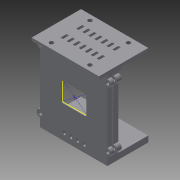
# Autodesk Inventor part: Nikon Base 02
Saved by Autodesk Inventor 2013 (Build 170138000, 138)
## iProperties
Created: 2014-04-13
Part Number: Nikon Base 02
Material: Generic
Document SubType Name: Modeling
Designer: spichelh
Density: 1 g/cm^3
Author: spichelh
Autodesk Inventor part; units mm, degrees
ref_plane "YZ Plane" through (0, 0, 0) normal (1, 0, 0) x (0, 1, 0)
ref_plane "XZ Plane" through (0, 0, 0) normal (0, 1, 0) x (-1, 0, 0)
ref_plane "XY Plane" through (0, 0, 0) normal (0, 0, 1) x (1, 0, 0)
sketch "Sketch1" plane through (0, 0, 0) normal (0, 0, 1) x (1, 0, 0)
  line L0 (55.88, 58.53) -> (0, 58.53)
  circle A0 centre (0, 3) radius 1.5
  arc A1 (0, 6) -> (0, 0) centre (0, 3) ccw
  circle A2 centre (0, 52.53) radius 1.5
  arc A3 (0, 55.53) -> (0, 49.53) centre (0, 52.53) ccw
  line L1 (27.94, 5) -> (27.94, 58.53) construction
  circle A4 centre (55.88, 3) radius 1.5
  arc A5 (55.88, 0) -> (55.88, 6) centre (55.88, 3) ccw
  circle A6 centre (55.88, 52.53) radius 1.5
  arc A7 (55.88, 49.53) -> (55.88, 55.53) centre (55.88, 52.53) ccw
  line L2 (55.88, 6) -> (55.88, 49.53)
  line L3 (55.88, 55.53) -> (55.88, 58.53)
  line L4 (0, 58.53) -> (0, 55.53)
  line L5 (0, 49.53) -> (0, 6)
  line L6 (52.88, 56.53) -> (3, 56.53)
  line L7 (0, 0) -> (0, 6) construction
  line L8 (55.88, 0) -> (55.88, 6) construction
  line L9 (0, 0) -> (0, -7)
  line L10 (0, -7) -> (55.88, -7)
  line L11 (55.88, -7) -> (55.88, 0)
  line L12 (50.88, 56.34) -> (5, 56.34) construction
  line L13 (3, -2.5) -> (52.88, -2.5)
  line L14 (3, 56.53) -> (3, -2.5)
  line L15 (52.88, -2.5) -> (52.88, 56.53)
  dimension "d0" = 55.88
  dimension "d2" = 3
  dimension "d3" = 6
  dimension "d4" = 3
  dimension "d5" = 6
  dimension "d6" = 49.53
  dimension "d8" = 3
  dimension "d14" = 2
  dimension "d16" = 7
  dimension "d17" = 7
  dimension "d78" = 3
  dimension "d79" = 3
  dimension "d214" = 4.5
  dimension "d215" = 3
  constraints: 30 end point, 9 parallel, 8 centre point, 8 point on circle, 5 coincident, 4 symmetric about line, 3 midpoint, 3 perpendicular, 1 collinear, 1 point on line, 4 other
  measures "d0" distance of L7.start L8.start
  measures "d2" diameter of A0
  measures "d3" diameter of A1
  measures "d4" diameter of A2
  measures "d5" diameter of A3
  measures "d6" distance of A0.centre A2.centre
  measures "d8" distance of A0.centre L7.start
  measures "d14" distance between parallel lines of L0 L6
  measures "d16" distance of L7.start L9.end
  measures "d17" distance of L10.end L8.start
  measures "d78" distance between parallel lines of L15 L2
  measures "d79" distance between parallel lines of L5 L14
  measures "d214" distance between parallel lines of L10 L13
  measures "d215" distance of L0.end L4.end
extrude "Extrusion1" add sketch "Sketch1" along normal blind 9
sketch "Sketch14" plane through (0, 0, 9) normal (0, 0, 1) x (1, 0, 0)
  line L0 (3, 56.53) -> (52.88, 56.53)
  line L1 (52.88, 56.53) -> (52.88, -2.5)
  line L2 (52.88, -2.5) -> (3, -2.5)
  line L3 (3, -2.5) -> (3, 56.53)
  circle A0 centre (27.94, 27.765) radius 23
  line L4 (27.94, 56.53) -> (27.94, -2.5) construction
  line L5 (50.88, 56.34) -> (5, 56.34) construction
  line L6 (-22.86, -0.81) -> (78.74, -0.81) construction
  line L7 (-22.86, 56.34) -> (-22.86, -0.81) construction
  line L8 (78.74, -0.81) -> (78.74, 56.34) construction
  line L9 (78.74, 27.765) -> (-22.86, 27.765) construction
  dimension "d96" = 46
  constraints: 12 end point, 5 midpoint, 2 parallel, 1 centre point, 1 horizontal, 1 perpendicular, 1 point on line
  measures "d96" diameter of A0
extrude "Extrusion14" add sketch "Sketch14" against normal blind 2
sketch "Sketch17" plane through (0, 0, 7) normal (0, 0, -1) x (-1, 0, 0)
  circle A0 centre (-27.94, 27.765) radius 23 construction
  line L0 (-37.34, 35.815) -> (-18.54, 35.815)
  line L1 (-17.54, 34.815) -> (-17.54, 20.715)
  line L2 (-18.54, 19.715) -> (-37.34, 19.715)
  line L3 (-38.34, 20.715) -> (-38.34, 34.815)
  line L4 (-17.54, 35.815) -> (-38.34, 19.715) construction
  line L5 (-17.54, 19.715) -> (-38.34, 35.815) construction
  circle A1 centre (-27.94, 27.765) radius 23
  arc A2 (-37.34, 35.815) -> (-38.34, 34.815) centre (-37.34, 34.815) ccw
  arc A3 (-38.34, 20.715) -> (-37.34, 19.715) centre (-37.34, 20.715) ccw
  arc A4 (-18.54, 19.715) -> (-17.54, 20.715) centre (-18.54, 20.715) ccw
  arc A5 (-17.54, 34.815) -> (-18.54, 35.815) centre (-18.54, 34.815) ccw
  point P0 (0, 0)
  dimension "d111" = 20.8
  dimension "d112" = 16.1
  dimension "d115" = 1
  constraints: 12 end point, 8 point on circle, 8 point on line, 8 tangent, 5 centre point, 4 equal radius, 2 midpoint, 2 parallel, 1 coincident, 1 horizontal, 1 perpendicular
  measures "d111" distance of L5.start L4.end
  measures "d112" distance of L4.start L5.start
  measures "d115" radius of A2
extrude "Extrusion17" add sketch "Sketch17" against normal blind 2
sketch "Sketch26" plane through (0, 6, 0) normal (-1, 0, 0) x (0, 0, 1)
  line L0 (0, 0) -> (0, 43.53) projected
  line L1 (-1, 50.34) -> (0, 50.34) construction
  line L2 (-1, -6.81) -> (0, -6.81) construction
  line L3 (4, -6.81) -> (6, -6.81)
  line L4 (6, -6.81) -> (6, 50.34)
  line L5 (6, 50.34) -> (4, 50.34)
  line L6 (4, 50.34) -> (4, -6.81)
  point P0 (0, -6)
  dimension "d140" = 2
  dimension "d141" = 4
  constraints: 8 end point, 2 collinear, 2 parallel, 1 horizontal, 1 perpendicular
  measures "d140" distance of L5.end L4.end
  measures "d141" distance between parallel lines of L0 L6
extrude "Extrusion26" cut sketch "Sketch26" along normal blind 3 and the other way blind 2
sketch "Sketch27" plane through (55.88, 6, 0) normal (1, 0, 0) x (0, 0, -1)
  line L0 (1, -6.81) -> (0, -6.81) construction
  line L1 (1, 50.34) -> (0, 50.34) construction
  line L2 (-4, 50.34) -> (-6, 50.34)
  line L3 (-6, 50.34) -> (-6, -6.81)
  line L4 (-6, -6.81) -> (-4, -6.81)
  line L5 (-4, -6.81) -> (-4, 50.34)
  line L6 (0, -6) -> (0, -13) construction
  dimension "d146" = 2
  dimension "d147" = 4
  constraints: 8 end point, 2 collinear, 2 parallel, 1 horizontal, 1 perpendicular
  measures "d146" distance of L4.end L3.end
  measures "d147" distance between parallel lines of L6 L5
extrude "Extrusion27" cut sketch "Sketch27" against normal blind 1.5 and the other way blind 3
sketch "Sketch32" plane through (0, 0, 0) normal (0, 0, -1) x (-1, 0, 0)
  line L0 (-55.88, -7) -> (0, -7)
  line L1 (0, -7) -> (0, -2)
  line L2 (0, -2) -> (-55.88, -2)
  line L3 (-55.88, -2) -> (-55.88, -7)
  dimension "d180" = 5
  dimension "d206" = 55.88
  constraints: 8 end point, 2 parallel, 1 horizontal, 1 perpendicular
  measures "d180" distance between parallel lines of L0 L2
  measures "d206" distance of L0.start L0.end
extrude "Extrusion32" add sketch "Sketch32" along normal blind 25 and the other way blind 1.5
sketch "Sketch35" plane through (0, -7, 9) normal (0, -1, 0) x (1, 0, 0)
  line L0 (55.88, -34) -> (0, -34) projected
  line L1 (0, -34) -> (55.88, 0) construction
  line L2 (55.88, -34) -> (0, 0) construction
  line L3 (27.94, -17) -> (27.94, -24.0701) construction
  circle A0 centre (27.94, -27) radius 3.175
  circle A1 centre (27.94, -15) radius 3.175
  point P0 (0, -9)
  dimension "d194" = 6.35
  dimension "d195" = 10
  dimension "d196" = 6.35
  dimension "d197" = 2
  constraints: 6 end point, 2 centre point, 2 point on line, 1 midpoint, 1 perpendicular
  measures "d194" diameter of A0
  measures "d195" distance of L3.start A0.centre
  measures "d196" diameter of A1
  measures "d197" distance of L3.start A1.centre
extrude "Extrusion34" cut sketch "Sketch35" against normal blind 10
sketch "Sketch37" plane through (52.88, -2, 0) normal (0, 1, 0) x (1, 0, 0)
  line L0 (-49.88, -1.5) -> (-49.88, 0) projected
  line L1 (0, -1.5) -> (-49.88, -1.5) projected
  line L2 (0, -1.5) -> (-49.88, -1.5)
  line L3 (-49.88, -1.5) -> (-49.88, 0)
  line L4 (-49.88, 0) -> (0, 0)
  line L5 (0, 0) -> (0, -1.5)
  constraints: 8 end point, 2 parallel, 1 horizontal, 1 perpendicular
extrude "Extrusion36" add sketch "Sketch37" along normal blind 3
sketch "Sketch38" plane through (0, 0, 7) normal (0, 0, -1) x (-1, 0, 0)
  arc A0 (-38.34, 20.715) -> (-37.34, 19.715) centre (-37.34, 20.715) ccw projected
  line L0 (-38.34, 20.715) -> (-38.34, 34.815) projected
  arc A1 (-37.34, 35.815) -> (-38.34, 34.815) centre (-37.34, 34.815) ccw projected
  line L1 (-37.34, 35.815) -> (-18.54, 35.815) projected
  arc A2 (-17.54, 34.815) -> (-18.54, 35.815) centre (-18.54, 34.815) ccw projected
  line L2 (-17.54, 34.815) -> (-17.54, 20.715) projected
  arc A3 (-18.54, 19.715) -> (-17.54, 20.715) centre (-18.54, 20.715) ccw projected
  line L3 (-18.54, 19.715) -> (-37.34, 19.715) projected
  line L4 (-18.54, 34.815) -> (-37.34, 20.715) construction
  line L5 (-18.54, 20.715) -> (-37.34, 34.815) construction
  line L6 (-45.055, 44.88) -> (-10.825, 44.88)
  line L7 (-10.825, 44.88) -> (-10.825, 10.65)
  line L8 (-10.825, 10.65) -> (-45.055, 10.65)
  line L9 (-45.055, 10.65) -> (-45.055, 44.88)
  line L10 (-10.825, 10.65) -> (-45.055, 44.88) construction
  line L11 (-45.055, 10.65) -> (-10.825, 44.88) construction
  point P0 (0, 0)
  point P1 (-27.94, 27.765)
  dimension "d209" = 34.23
  dimension "d211" = 34.23
  constraints: 16 end point, 3 midpoint, 2 parallel, 1 horizontal, 1 perpendicular
  measures "d209" distance of L8.end L6.start
  measures "d211" distance of L6.start L6.end
extrude "Extrusion37" cut sketch "Sketch38" against normal blind 1
sketch "Sketch39" plane through (0, 0, 8) normal (0, 0, -1) x (-1, 0, 0)
  line L0 (-37.34, 19.715) -> (-18.54, 19.715) projected
  arc A0 (-38.34, 20.715) -> (-37.34, 19.715) centre (-37.34, 20.715) ccw projected
  line L1 (-38.34, 34.815) -> (-38.34, 20.715) projected
  arc A1 (-37.34, 35.815) -> (-38.34, 34.815) centre (-37.34, 34.815) ccw projected
  line L2 (-18.54, 35.815) -> (-37.34, 35.815) projected
  arc A2 (-17.54, 34.815) -> (-18.54, 35.815) centre (-18.54, 34.815) ccw projected
  line L3 (-17.54, 20.715) -> (-17.54, 34.815) projected
  arc A3 (-18.54, 19.715) -> (-17.54, 20.715) centre (-18.54, 20.715) ccw projected
  line L4 (-45.055, 44.88) -> (-10.825, 44.88) projected
  line L5 (-45.055, 10.65) -> (-45.055, 44.88) projected
  line L6 (-10.825, 10.65) -> (-45.055, 10.65) projected
  line L7 (-10.825, 44.88) -> (-10.825, 10.65) projected
  line L8 (-18.54, 34.815) -> (-37.34, 20.715) construction
  line L9 (-37.34, 34.815) -> (-18.54, 20.715) construction
  point P0 (0, 0)
  point P1 (-27.94, 27.765)
  constraints: 4 end point, 1 midpoint
sketch "Sketch40" plane through (0, 0, 9) normal (0, 0, 1) x (1, 0, 0)
  line L0 (0, 58.53) -> (55.88, 58.53)
  line L1 (55.88, 58.53) -> (55.88, 61.03)
  line L2 (55.88, 61.03) -> (0, 61.03)
  line L3 (0, 61.03) -> (0, 58.53)
  dimension "d216" = 2.5
  dimension "d217" = 55.88
  constraints: 8 end point, 2 parallel, 1 horizontal, 1 perpendicular
  measures "d216" distance of L2.end L0.start
  measures "d217" distance between parallel lines of L3 L1
extrude "Extrusion38" add sketch "Sketch40" along normal blind 7 and the other way blind 34
sketch "Sketch43" plane through (0, 61.03, 16) normal (0, 1, 0) x (1, 0, 0)
  line L0 (52.88, 24) -> (3, 24)
  line L1 (3, 29) -> (3, 24)
  line L2 (52.88, 29) -> (3, 29)
  line L3 (52.88, 29) -> (52.88, 24)
  line L4 (12, 30) -> (14, 30)
  line L5 (14, 30) -> (14, 25)
  line L6 (14, 25) -> (12, 25)
  line L7 (12, 25) -> (12, 30)
  line L8 (17, 30) -> (19, 30)
  line L9 (19, 30) -> (19, 25)
  line L10 (19, 25) -> (17, 25)
  line L11 (17, 25) -> (17, 30)
  line L12 (22, 30) -> (24, 30)
  line L13 (24, 30) -> (24, 25)
  line L14 (24, 25) -> (22, 25)
  line L15 (22, 25) -> (22, 30)
  line L16 (27, 30) -> (29, 30)
  line L17 (29, 30) -> (29, 25)
  line L18 (29, 25) -> (27, 25)
  line L19 (27, 25) -> (27, 30)
  line L20 (32, 30) -> (34, 30)
  line L21 (34, 30) -> (34, 25)
  line L22 (34, 25) -> (32, 25)
  line L23 (32, 25) -> (32, 30)
  line L24 (37, 30) -> (39, 30)
  line L25 (39, 30) -> (39, 25)
  line L26 (39, 25) -> (37, 25)
  line L27 (37, 25) -> (37, 30)
  line L28 (42, 30) -> (44, 30)
  line L29 (44, 30) -> (44, 25)
  line L30 (44, 25) -> (42, 25)
  line L31 (42, 25) -> (42, 30)
  line L32 (0, 41) -> (0, 0) projected
  line L33 (55.88, 41) -> (55.88, 0) projected
  line L34 (0, 21) -> (55.88, 21) construction
  line L35 (12, 12) -> (14, 12)
  line L36 (14, 12) -> (14, 17)
  line L37 (14, 17) -> (12, 17)
  line L38 (12, 17) -> (12, 12)
  line L39 (19, 12) -> (19, 17)
  line L40 (17, 12) -> (19, 12)
  line L41 (19, 17) -> (17, 17)
  line L42 (24, 12) -> (24, 17)
  line L43 (22, 12) -> (24, 12)
  line L44 (22, 17) -> (22, 12)
  line L45 (24, 17) -> (22, 17)
  line L46 (29, 12) -> (29, 17)
  line L47 (27, 12) -> (29, 12)
  line L48 (27, 17) -> (27, 12)
  line L49 (29, 17) -> (27, 17)
  line L50 (34, 12) -> (34, 17)
  line L51 (32, 12) -> (34, 12)
  line L52 (32, 17) -> (32, 12)
  line L53 (34, 17) -> (32, 17)
  line L54 (39, 12) -> (39, 17)
  line L55 (37, 12) -> (39, 12)
  line L56 (37, 17) -> (37, 12)
  line L57 (39, 17) -> (37, 17)
  line L58 (44, 12) -> (44, 17)
  line L59 (42, 12) -> (44, 12)
  line L60 (42, 17) -> (42, 12)
  line L61 (44, 17) -> (42, 17)
  line L62 (17, 17) -> (17, 12)
  line L63 (55.88, 0) -> (0, 0) projected
  point P0 (0, 27)
  dimension "d233" = 1
  dimension "d234" = 1
  dimension "d235" = 2
  dimension "d236" = 9
  dimension "d239" = 5
  dimension "d295" = 3
  dimension "d296" = 3
  dimension "d297" = 8.88
  dimension "d298" = 5
  dimension "d299" = 21
  constraints: 122 end point, 28 symmetric about line, 2 horizontal, 2 parallel, 2 perpendicular, 2 point on line, 48 other
  measures "d233" distance between parallel lines of L2 L4
  measures "d234" distance between parallel lines of L0 L6
  measures "d235" distance between parallel lines of L7 L5
  measures "d236" distance between parallel lines of L7 L1
  measures "d239" distance of L4.end L9.start
  measures "d295" distance between parallel lines of L32 L1
  measures "d296" distance between parallel lines of L33 L3
  measures "d297" distance between parallel lines of L3 L29
  measures "d298" distance between parallel lines of L8 L10
  measures "d299" distance between parallel lines of L63 L34
extrude "Extrusion41" cut sketch "Sketch43" against normal blind 5 contours L29 L30 L31 L2 | L2 L31 L28 L29 | L7 L4 L5 L2 | L2 L5 L6 L7 | L25 L26 L27 L2 | L2 L27 L24 L25 | L11 L8 L9 L2 | L2 L9 L10 L11 | L21 L22 L23 L2 | L2 L23 L20 L21 | L15 L12 L13 L2 | L2 L13 L14 L15 | L17 L18 L19 L2 | L2 L19 L16 L17 | L38 L37 L36 L35 | L40 L62 L41 L39 | L43 L44 L45 L42 | L47 L48 L49 L46 | L51 L52 L53 L50 | L55 L56 L57 L54 | L59 L60 L61 L58
sketch "Sketch44" plane through (0, -7, 9) normal (0, -1, 0) x (1, 0, 0)
  line L0 (52.88, -7.5) -> (3, -7.5) projected
  line L1 (3, -7.5) -> (3, -2) projected
  line L2 (3, -2) -> (52.88, -2) projected
  line L3 (52.88, -7.5) -> (52.88, -2) projected
  line L4 (5, -3) -> (7, -3)
  line L5 (7, -3) -> (7, -6.5)
  line L6 (7, -6.5) -> (5, -6.5)
  line L7 (5, -6.5) -> (5, -3)
  line L8 (10.5, -3) -> (12.5, -3)
  line L9 (12.5, -3) -> (12.5, -6.5)
  line L10 (12.5, -6.5) -> (10.5, -6.5)
  line L11 (10.5, -6.5) -> (10.5, -3)
  line L12 (16, -3) -> (18, -3)
  line L13 (18, -3) -> (18, -6.5)
  line L14 (18, -6.5) -> (16, -6.5)
  line L15 (16, -6.5) -> (16, -3)
  line L16 (21.5, -3) -> (23.5, -3)
  line L17 (23.5, -3) -> (23.5, -6.5)
  line L18 (23.5, -6.5) -> (21.5, -6.5)
  line L19 (21.5, -6.5) -> (21.5, -3)
  line L20 (27, -3) -> (29, -3)
  line L21 (29, -3) -> (29, -6.5)
  line L22 (29, -6.5) -> (27, -6.5)
  line L23 (27, -6.5) -> (27, -3)
  line L24 (32.5, -3) -> (34.5, -3)
  line L25 (34.5, -3) -> (34.5, -6.5)
  line L26 (34.5, -6.5) -> (32.5, -6.5)
  line L27 (32.5, -6.5) -> (32.5, -3)
  line L28 (38, -3) -> (40, -3)
  line L29 (40, -3) -> (40, -6.5)
  line L30 (40, -6.5) -> (38, -6.5)
  line L31 (38, -6.5) -> (38, -3)
  line L32 (43.5, -3) -> (45.5, -3)
  line L33 (45.5, -3) -> (45.5, -6.5)
  line L34 (45.5, -6.5) -> (43.5, -6.5)
  line L35 (43.5, -6.5) -> (43.5, -3)
  line L36 (49, -3) -> (51, -3)
  line L37 (51, -3) -> (51, -6.5)
  line L38 (51, -6.5) -> (49, -6.5)
  line L39 (49, -6.5) -> (49, -3)
  point P0 (0, -9)
  dimension "d247" = 1
  dimension "d248" = 1
  dimension "d249" = 2
  dimension "d250" = 2
  dimension "d253" = 5.5
  dimension "d260" = 1.88
  constraints: 72 end point, 2 horizontal, 2 parallel, 1 perpendicular, 64 other
  measures "d247" distance between parallel lines of L2 L4
  measures "d248" distance between parallel lines of L0 L6
  measures "d249" distance between parallel lines of L7 L5
  measures "d250" distance between parallel lines of L1 L7
  measures "d253" distance of L4.end L9.start
  measures "d260" distance between parallel lines of L37 L3
extrude "Extrusion42" cut sketch "Sketch44" against normal blind 5 contours L4 L5 L6 L7 | L8 L9 L10 L11 | L12 L13 L14 L15 | L16 L17 L18 L19 | L20 L21 L22 L23 | L24 L25 L26 L27 | L28 L29 L30 L31 | L32 L33 L34 L35 | L36 L37 L38 L39
sketch "Sketch46" plane through (0, 61.03, 16) normal (0, 1, 0) x (1, 0, 0)
  circle A0 centre (11.94, 36.5) radius 1.7
  circle A1 centre (43.94, 36.5) radius 1.7
  line L0 (43.94, 36.5) -> (11.94, 36.5) construction
  circle A2 centre (43.94, 4.5) radius 1.7
  line L1 (0, 41) -> (0, 0) projected
  line L2 (55.88, 0) -> (0, 0) projected
  line L3 (55.88, 41) -> (55.88, 0) projected
  line L4 (0, 41) -> (55.88, 41) projected
  line L5 (55.88, 20.5) -> (0, 20.5) construction
  line L6 (27.94, 41) -> (27.94, 0) construction
  line L7 (49, 21) -> (47, 21) projected
  line L8 (43.94, 4.5) -> (43.94, 36.5) construction
  circle A3 centre (11.94, 4.5) radius 1.7
  point P0 (27.94, 36.5)
  point P1 (43.94, 20.5)
  dimension "d275" = 3.4
  dimension "d277" = 3.4
  dimension "d278" = 32
  dimension "d279" = 32
  dimension "d294" = 3.4
  constraints: 8 end point, 6 midpoint, 4 centre point, 2 point on line, 1 horizontal, 1 perpendicular, 1 symmetric about line, 1 other
  measures "d275" diameter of A0
  measures "d277" diameter of A1
  measures "d278" distance of L0.start L0.end
  measures "d279" distance of L8.start L0.start
  measures "d294" diameter of A2
extrude "Extrusion44" cut sketch "Sketch46" against normal blind 5 contours A0 | A1 | A2 | A3
sketch "Sketch48" plane through (3, 56.53, 0) normal (0, -1, 0) x (1, 0, 0)
  line L0 (0, 0) -> (0, 7) projected
  line L1 (49.88, 0) -> (0, 0) projected
  line L2 (1, 0) -> (49, 0)
  line L3 (49, 0) -> (49, 4)
  line L4 (49, 4) -> (1, 4)
  line L5 (1, 4) -> (1, 0)
  point P0 (-3, 0)
  dimension "d282" = 4
  dimension "d284" = 48
  dimension "d285" = 1
  constraints: 8 end point, 2 parallel, 1 horizontal, 1 perpendicular, 1 point on line
  measures "d282" distance between parallel lines of L2 L4
  measures "d284" distance between parallel lines of L3 L5
  measures "d285" distance between parallel lines of L0 L5
extrude "Extrusion45" cut sketch "Sketch48" against normal blind 2
sketch "Sketch49" plane through (0, 0, 0) normal (0, 0, -1) x (-1, 0, 0)
  line L0 (0, 55.53) -> (0, 58.53) projected
  line L1 (-55.88, 58.53) -> (0, 58.53)
  line L2 (0, 58.53) -> (0, 56.53)
  line L3 (0, 56.53) -> (-55.88, 56.53)
  line L4 (-55.88, 56.53) -> (-55.88, 58.53)
  constraints: 8 end point, 2 parallel, 1 horizontal, 1 perpendicular, 1 point on line
extrude "Extrusion46" add sketch "Sketch49" along normal blind 2
sketch "Sketch50" plane through (0, 61.03, 16) normal (0, 1, 0) x (1, 0, 0)
  line L0 (2.5, 2.5) -> (2.5, 37.5) projected
  line L1 (2.5, 37.5) -> (53.38, 37.5) projected
  line L2 (53.38, 37.5) -> (53.38, 2.5) projected
  line L3 (53.38, 2.5) -> (2.5, 2.5) projected
  line L4 (0, 41) -> (0, 0) projected
  line L5 (55.88, 0) -> (0, 0) projected
  line L6 (0, 41) -> (55.88, 41)
  line L7 (55.88, 41) -> (55.88, 0)
  line L8 (55.88, 0) -> (0, 0)
  line L9 (0, 0) -> (0, 41)
  point P0 (0, 16)
  constraints: 8 end point, 2 parallel, 1 horizontal, 1 perpendicular
extrude "Extrusion47" [suppressed]
sketch "Sketch51" plane through (0, 0, 7) normal (0, 0, -1) x (-1, 0, 0)
  line L0 (-10.825, 10.65) -> (-45.055, 10.65) projected
  line L1 (-3, -2.5) -> (-52.88, -2.5) projected
  line L2 (-37.44, -2.5) -> (-35.44, -2.5)
  line L3 (-35.44, -2.5) -> (-35.44, 0.5)
  line L4 (-35.44, 0.5) -> (-37.44, 0.5)
  line L5 (-37.44, 0.5) -> (-37.44, -2.5)
  line L6 (-27.94, -2.5) -> (-27.94, 10.65) construction
  line L7 (-31.94, -2.5) -> (-29.94, -2.5)
  line L8 (-29.94, -2.5) -> (-29.94, 0.5)
  line L9 (-29.94, 0.5) -> (-31.94, 0.5)
  line L10 (-31.94, 0.5) -> (-31.94, -2.5)
  line L11 (-26.44, -2.5) -> (-24.44, -2.5)
  line L12 (-24.44, -2.5) -> (-24.44, 0.5)
  line L13 (-24.44, 0.5) -> (-26.44, 0.5)
  line L14 (-26.44, 0.5) -> (-26.44, -2.5)
  line L15 (-20.94, -2.5) -> (-18.94, -2.5)
  line L16 (-18.94, -2.5) -> (-18.94, 0.5)
  line L17 (-18.94, 0.5) -> (-20.94, 0.5)
  line L18 (-20.94, 0.5) -> (-20.94, -2.5)
  point P0 (0, 0)
  dimension "d300" = 0
  dimension "d301" = 2
  dimension "d302" = 3
  dimension "d303" = 15
  dimension "d308" = 5.5
  constraints: 34 end point, 2 horizontal, 2 midpoint, 2 parallel, 1 perpendicular, 24 other
  measures "d300" distance between parallel lines of L2 L1
  measures "d301" distance of L2.start L2.end
  measures "d302" distance between parallel lines of L4 L2
  measures "d303" diameter of L3 L6
  measures "d308" distance of L3.end L9.start
extrude "Extrusion48" cut sketch "Sketch51" against normal blind 10
body "Solid1"
